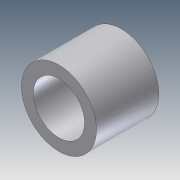
# Autodesk Inventor part: PP-00043
Saved by Autodesk Inventor 2012 (Build 160160000, 160)
## iProperties
Created: 2011-11-20
Part Number: PP-00043
Document SubType Name: Modeling
Designer: dfoster
Density: 1 g/cm^3
Description: Spacer, Aluminum
Material: Default
Title: Spacer, Aluminum
Author: dfoster
Autodesk Inventor part; units mm, degrees
ref_plane "YZ Plane" through (0, 0, 0) normal (1, 0, 0) x (0, 1, 0)
ref_plane "XZ Plane" through (0, 0, 0) normal (0, 1, 0) x (-1, 0, 0)
ref_plane "XY Plane" through (0, 0, 0) normal (0, 0, 1) x (1, 0, 0)
sketch "Sketch1" plane through (0, 0, 0) normal (0, 0, 1) x (1, 0, 0)
  circle A0 centre (0, 0) radius 4.7625
  circle A1 centre (0, 0) radius 3.2639
  dimension "d0" = 9.525
  dimension "d1" = 6.5278
  constraints: 2 centre point, 2 coincident
  measures "d0" diameter of A0
  measures "d1" diameter of A1
extrude "Extrusion1" add sketch "Sketch1" along normal blind 7.9375
body "Solid1"
